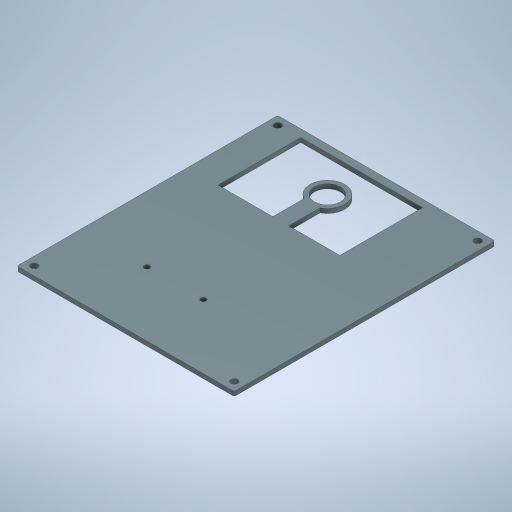
# Autodesk Inventor part: bevel desk (hole)
Saved by Autodesk Inventor 2024 (Build 280153000, 153)
## iProperties
Created: 2023-06-07
Part Number: bevel desk (hole)
Material: Lead
Document SubType Name: Modeling
Designer: shraa
Density: 11.34 g/cm^3
Appearance: Lead
Author: shraa
Autodesk Inventor part; units mm, degrees
ref_plane "YZ Plane" through (0, 0, 0) normal (1, 0, 0) x (0, 1, 0)
ref_plane "XZ Plane" through (0, 0, 0) normal (0, 1, 0) x (-1, 0, 0)
ref_plane "XY Plane" through (0, 0, 0) normal (0, 0, 1) x (1, 0, 0)
sketch "Sketch2" plane through (0, 0, 0) normal (0, 1, 0) x (-1, 0, 0)
  line L0 (0, 0) -> (250, 0)
  line L1 (250, 0) -> (250, -300)
  line L2 (250, -300) -> (0, -300)
  line L3 (0, -300) -> (0, 0)
  dimension "d4" = 250
  dimension "d5" = 300
  constraints: 8 end point, 2 parallel, 1 horizontal, 1 perpendicular
  measures "d4" distance of L1.end L2.end
  measures "d5" distance of L0.end L1.end
extrude "Extrusion2" add sketch "Sketch2" along normal blind 5
fillet "Fillet1" radius 2 4 edges at (0, 2.5, 0) (-250, 2.5, 0) (-250, 2.5, -300) (0, 2.5, -300)
sketch "Sketch5" plane through (0, 5, 0) normal (0, 1, 0) x (1, 0, 0)
  line L0 (-2, 300) -> (-248, 300) projected
  circle A0 centre (-10, 10) radius 5 projected
  circle A1 centre (-10, 290) radius 5 projected
  circle A2 centre (-240, 290) radius 5 projected
  circle A3 centre (-240, 10) radius 5 projected
  point P0 (0, 0)
  point P1 (-15, 150)
  dimension "d25" = 150
  constraints: 4 coincident
  measures "d25" distance from line of L0 point (-15, 150)
hole "Hole1" at (-240, 5, -10) at (-10, 5, -10) at (-10, 5, -290) at (-240, 5, -290) direction (0, -1, 0) diameter 8 depth 25 tip angle 118
sketch "Sketch6" plane through (0, 5, 0) normal (0, 1, 0) x (1, 0, 0)
  circle A0 centre (-142.8286, 250) radius 15
  line L0 (-2, 300) -> (-248, 300) projected
  circle A1 centre (-142.8286, 250) radius 20
  line L1 (-133.6124, 232.25) -> (-133.6124, 196.3478)
  line L2 (-152.0448, 232.25) -> (-152.0448, 196.3478)
  line L3 (-214.8824, 196.3478) -> (-74.8824, 196.3478)
  line L4 (-74.8824, 196.3478) -> (-74.8824, 291.3478)
  line L5 (-74.8824, 291.3478) -> (-214.8824, 291.3478)
  line L6 (-214.8824, 291.3478) -> (-214.8824, 196.3478)
  point P0 (0, 0)
  dimension "d33" = 30
  dimension "d34" = 50
  dimension "d35" = 40
  dimension "d36" = 140
  dimension "d37" = 95
  constraints: 12 end point, 2 centre point, 2 parallel, 2 point on circle, 2 vertical, 1 coincident, 1 horizontal, 1 perpendicular
  measures "d33" diameter of A0
  measures "d34" distance from line of L0 A0.centre
  measures "d35" diameter of A1
  measures "d36" distance of L5.end L4.end
  measures "d37" distance of L4.end L3.end
extrude "Extrusion5" cut sketch "Sketch6" against normal blind 50 contours A0 | A1 L2 L3 L6 L5 L4 L1
sketch "Sketch8" plane through (0, 5, 0) normal (0, 1, 0) x (1, 0, 0)
  line L0 (-152.0448, 196.3478) -> (-214.8824, 196.3478) projected
  line L1 (-133.6124, 196.3478) -> (-74.8824, 196.3478) projected
  point P0 (0, 0)
  point P1 (-174.2431, 196.3478)
  point P2 (-174.3182, 73.8636)
  point P3 (-109.2711, 196.3478)
  point P4 (-109.3182, 73.8636)
  dimension "d47" = 65
  constraints: 2 point on line
  measures "d47" distance of point (-109.318, 73.864) point (-174.318, 73.864)
hole "Hole3" at (-174.3182, 5, -73.8636) at (-109.3182, 5, -73.8636) direction (0, -1, 0) diameter 6 depth 25 tip angle 118
body "Solid2"
